Autodesk Fusion 360 part; units mm, degrees
(part 8 of 8)
  spline S41 degree 5 poles (20.6515, -12.2277) (20.6495, -12.2245) (20.6456, -12.2182) (20.6397, -12.2087) (20.6318, -12.1961) (20.6219, -12.1805) (20.6121, -12.1648) (20.6022, -12.1492) (20.5923, -12.1337) (20.5824, -12.1182) (20.5725, -12.1028) (20.5626, -12.0874) (20.5527, -12.0721) (20.5428, -12.0568) (20.5329, -12.0416) (20.523, -12.0264) (20.5131, -12.0112) (20.5032, -11.9962) (20.4932, -11.9811) (20.4833, -11.9661) (20.4734, -11.9512) (20.4634, -11.9363) (20.4535, -11.9215) (20.4436, -11.9067) (20.4336, -11.892) (20.4237, -11.8773) (20.4137, -11.8627) (20.4038, -11.8482) (20.3938, -11.8336) (20.3839, -11.8192) (20.3739, -11.8048) (20.364, -11.7904) (20.354, -11.7761) (20.3441, -11.7618) (20.3341, -11.7476) (20.3242, -11.7335) (20.3142, -11.7194) (20.3042, -11.7053) (20.2943, -11.6913) (20.2843, -11.6774) (20.2744, -11.6635) (20.2644, -11.6497) (20.2545, -11.6359) (20.2445, -11.6221) (20.2346, -11.6085) (20.2246, -11.5948) (20.2147, -11.5813) (20.2047, -11.5677) (20.1948, -11.5543) (20.1848, -11.5409) (20.1749, -11.5275) (20.165, -11.5142) (20.155, -11.501) (20.1451, -11.4878) (20.1352, -11.4746) (20.1253, -11.4615) (20.1154, -11.4485) (20.1054, -11.4355) (20.0955, -11.4226) (20.0856, -11.4097) (20.0757, -11.3969) (20.0659, -11.3842) (20.056, -11.3715) (20.0461, -11.3588) (20.0362, -11.3462) (20.0263, -11.3337) (20.0165, -11.3212) (20.0066, -11.3088) (19.9968, -11.2964) (19.9869, -11.2841) (19.9771, -11.2718) (19.9673, -11.2596) (19.9575, -11.2475) (19.9477, -11.2354) (19.9379, -11.2233) (19.9281, -11.2113) (19.9183, -11.1994) (19.9085, -11.1875) (19.8987, -11.1757) (19.889, -11.164) (19.8792, -11.1523) (19.8695, -11.1406) (19.8598, -11.1291) (19.8501, -11.1175) (19.8404, -11.1061) (19.8307, -11.0946) (19.821, -11.0833) (19.8113, -11.072) (19.8017, -11.0607) (19.7921, -11.0496) (19.7824, -11.0384) (19.7728, -11.0274) (19.7632, -11.0164) (19.7536, -11.0054) (19.7441, -10.9945) (19.7345, -10.9837) (19.725, -10.9729) (19.7154, -10.9622) (19.7059, -10.9515) (19.6964, -10.9409) (19.6869, -10.9304) (19.6775, -10.9199) (19.668, -10.9095) (19.6586, -10.8991) (19.6492, -10.8888) (19.6398, -10.8786) (19.6304, -10.8684) (19.621, -10.8583) (19.6117, -10.8482) (19.6024, -10.8382) (19.5931, -10.8282) (19.5838, -10.8184) (19.5745, -10.8085) (19.5653, -10.7988) (19.5561, -10.7891) (19.5469, -10.7794) (19.5377, -10.7698) (19.5285, -10.7603) (19.5194, -10.7509) (19.5103, -10.7415) (19.5012, -10.7321) (19.4921, -10.7229) (19.4831, -10.7136) (19.4741, -10.7045) (19.4651, -10.6954) (19.4561, -10.6864) (19.4472, -10.6774) (19.4382, -10.6685) (19.4293, -10.6596) (19.4205, -10.6509) (19.4116, -10.6421) (19.4028, -10.6335) (19.3941, -10.6249) (19.3853, -10.6164) (19.3766, -10.6079) (19.3679, -10.5995) (19.3592, -10.5912) (19.3506, -10.5829) (19.342, -10.5747) (19.3334, -10.5665) (19.3249, -10.5584) (19.3163, -10.5504) (19.3079, -10.5425) (19.2994, -10.5346) (19.291, -10.5267) (19.2826, -10.519) (19.2743, -10.5113) (19.266, -10.5036) (19.2577, -10.4961) (19.2495, -10.4886) (19.2413, -10.4811) (19.2331, -10.4738) (19.225, -10.4665) (19.2169, -10.4592) (19.2088, -10.452) (19.2008, -10.4449) (19.1929, -10.4379) (19.1849, -10.4309) (19.177, -10.424) (19.1692, -10.4172) (19.1614, -10.4104) (19.1536, -10.4037) (19.1459, -10.397) (19.1382, -10.3905) (19.1306, -10.384) (19.123, -10.3775) (19.1155, -10.3712) (19.108, -10.3649) (19.1006, -10.3586) (19.0932, -10.3525) (19.0858, -10.3464) (19.0785, -10.3403) (19.0713, -10.3344) (19.0641, -10.3285) (19.0569, -10.3227) (19.0498, -10.3169) (19.0428, -10.3112) (19.0358, -10.3056) (19.0289, -10.3001) (19.022, -10.2946) (19.0152, -10.2892) (19.0085, -10.2839) (19.0017, -10.2786) (18.9951, -10.2735) (18.9885, -10.2683) (18.982, -10.2633) (18.9755, -10.2583) (18.9691, -10.2534) (18.9628, -10.2486) (18.9565, -10.2439) (18.9503, -10.2392) (18.9442, -10.2346) (18.9381, -10.23) (18.9321, -10.2256) (18.9262, -10.2212) (18.9203, -10.2169) (18.9145, -10.2127) (18.9088, -10.2085) (18.9032, -10.2044) (18.8976, -10.2004) (18.8921, -10.1965) (18.8867, -10.1926) (18.8814, -10.1888) (18.8761, -10.1851) (18.8709, -10.1815) (18.8658, -10.1779) (18.8608, -10.1745) (18.8559, -10.1711) (18.8511, -10.1677) (18.8463, -10.1645) (18.8417, -10.1613) (18.8371, -10.1583) (18.8326, -10.1553) (18.8282, -10.1523) (18.824, -10.1495) (18.8198, -10.1467) (18.8157, -10.144) (18.8117, -10.1414) (18.8078, -10.1389) (18.804, -10.1365) (18.8003, -10.1341) (18.7968, -10.1319) (18.7933, -10.1297) (18.79, -10.1276) (18.7868, -10.1256) (18.7836, -10.1236) (18.7807, -10.1218) (18.7778, -10.12) (18.775, -10.1183) (18.7724, -10.1168) (18.7699, -10.1153) (18.7676, -10.1138) (18.7654, -10.1125) (18.7633, -10.1113) (18.7613, -10.1102) (18.7595, -10.1091) (18.7579, -10.1081) (18.7564, -10.1073) (18.755, -10.1065) (18.7538, -10.1058) (18.7528, -10.1053) (18.7521, -10.1049) (18.7517, -10.1046) (18.7514, -10.1045) (18.7513, -10.1044) knots -1 -1 -1 -1 -1 -1 -0.99583333 -0.99166667 -0.9875 -0.98333333 -0.97916667 -0.975 -0.97083333 -0.96666667 -0.9625 -0.95833333 -0.95416667 -0.95 -0.94583333 -0.94166667 -0.9375 -0.93333333 -0.92916667 -0.925 -0.92083333 -0.91666667 -0.9125 -0.90833333 -0.90416667 -0.9 -0.89583333 -0.89166667 -0.8875 -0.88333333 -0.87916667 -0.875 -0.87083333 -0.86666667 -0.8625 -0.85833333 -0.85416667 -0.85 -0.84583333 -0.84166667 -0.8375 -0.83333333 -0.82916667 -0.825 -0.82083333 -0.81666667 -0.8125 -0.80833333 -0.80416667 -0.8 -0.79583333 -0.79166667 -0.7875 -0.78333333 -0.77916667 -0.775 -0.77083333 -0.76666667 -0.7625 -0.75833333 -0.75416667 -0.75 -0.74583333 -0.74166667 -0.7375 -0.73333333 -0.72916667 -0.725 -0.72083333 -0.71666667 -0.7125 -0.70833333 -0.70416667 -0.7 -0.69583333 -0.69166667 -0.6875 -0.68333333 -0.67916667 -0.675 -0.67083333 -0.66666667 -0.6625 -0.65833333 -0.65416667 -0.65 -0.64583333 -0.64166667 -0.6375 -0.63333333 -0.62916667 -0.625 -0.62083333 -0.61666667 -0.6125 -0.60833333 -0.60416667 -0.6 -0.59583333 -0.59166667 -0.5875 -0.58333333 -0.57916667 -0.575 -0.57083333 -0.56666667 -0.5625 -0.55833333 -0.55416667 -0.55 -0.54583333 -0.54166667 -0.5375 -0.53333333 -0.52916667 -0.525 -0.52083333 -0.51666667 -0.5125 -0.50833333 -0.50416667 -0.5 -0.49583333 -0.49166667 -0.4875 -0.48333333 -0.47916667 -0.475 -0.47083333 -0.46666667 -0.4625 -0.45833333 -0.45416667 -0.45 -0.44583333 -0.44166667 -0.4375 -0.43333333 -0.42916667 -0.425 -0.42083333 -0.41666667 -0.4125 -0.40833333 -0.40416667 -0.4 -0.39583333 -0.39166667 -0.3875 -0.38333333 -0.37916667 -0.375 -0.37083333 -0.36666667 -0.3625 -0.35833333 -0.35416667 -0.35 -0.34583333 -0.34166667 -0.3375 -0.33333333 -0.32916667 -0.325 -0.32083333 -0.31666667 -0.3125 -0.30833333 -0.30416667 -0.3 -0.29583333 -0.29166667 -0.2875 -0.28333333 -0.27916667 -0.275 -0.27083333 -0.26666667 -0.2625 -0.25833333 -0.25416667 -0.25 -0.24583333 -0.24166667 -0.2375 -0.23333333 -0.22916667 -0.225 -0.22083333 -0.21666667 -0.2125 -0.20833333 -0.20416667 -0.2 -0.19583333 -0.19166667 -0.1875 -0.18333333 -0.17916667 -0.175 -0.17083333 -0.16666667 -0.1625 -0.15833333 -0.15416667 -0.15 -0.14583333 -0.14166667 -0.1375 -0.13333333 -0.12916667 -0.125 -0.12083333 -0.11666667 -0.1125 -0.10833333 -0.10416667 -0.1 -0.09583333 -0.09166667 -0.0875 -0.08333333 -0.07916667 -0.075 -0.07083333 -0.06666667 -0.0625 -0.05833333 -0.05416667 -0.05 -0.04583333 -0.04166667 -0.0375 -0.03333333 -0.02916667 -0.025 -0.02083333 -0.01666667 -0.0125 -0.00833333 -0.00416667 0 0 0 0 0 0
  line L82 (18.7513, -10.1044) -> (18.7502, -10.1038)
  line L83 (18.7502, -10.1038) -> (17.1663, -9.2503)
  arc A42 (17.1663, -9.2503) -> (18.2325, -6.9158) centre (0, 0) ccw
  line L84 (18.2325, -6.9158) -> (19.9147, -7.5539)
  line L85 (19.9147, -7.5539) -> (19.9159, -7.5543)
  spline S42 degree 5 poles (19.9159, -7.5543) (19.916, -7.5543) (19.9163, -7.5544) (19.9168, -7.5546) (19.9175, -7.5549) (19.9186, -7.5553) (19.9199, -7.5557) (19.9214, -7.5563) (19.923, -7.5568) (19.9248, -7.5574) (19.9268, -7.5581) (19.9289, -7.5588) (19.9312, -7.5596) (19.9337, -7.5604) (19.9363, -7.5613) (19.9391, -7.5622) (19.942, -7.5631) (19.945, -7.5641) (19.9482, -7.5651) (19.9516, -7.5662) (19.9551, -7.5673) (19.9587, -7.5684) (19.9625, -7.5695) (19.9664, -7.5707) (19.9705, -7.5719) (19.9747, -7.5731) (19.979, -7.5744) (19.9834, -7.5757) (19.988, -7.577) (19.9927, -7.5783) (19.9975, -7.5797) (20.0025, -7.5811) (20.0076, -7.5825) (20.0128, -7.5839) (20.0181, -7.5853) (20.0235, -7.5868) (20.0291, -7.5882) (20.0348, -7.5897) (20.0406, -7.5912) (20.0465, -7.5927) (20.0525, -7.5942) (20.0586, -7.5958) (20.0649, -7.5973) (20.0712, -7.5989) (20.0777, -7.6004) (20.0843, -7.602) (20.0909, -7.6036) (20.0977, -7.6052) (20.1046, -7.6068) (20.1116, -7.6084) (20.1187, -7.61) (20.1259, -7.6116) (20.1332, -7.6132) (20.1406, -7.6148) (20.1481, -7.6165) (20.1557, -7.6181) (20.1634, -7.6197) (20.1712, -7.6213) (20.1791, -7.623) (20.1871, -7.6246) (20.1951, -7.6262) (20.2033, -7.6279) (20.2116, -7.6295) (20.2199, -7.6311) (20.2284, -7.6327) (20.2369, -7.6343) (20.2456, -7.636) (20.2543, -7.6376) (20.2631, -7.6392) (20.272, -7.6408) (20.281, -7.6424) (20.2901, -7.644) (20.2992, -7.6455) (20.3085, -7.6471) (20.3178, -7.6487) (20.3272, -7.6502) (20.3367, -7.6518) (20.3463, -7.6533) (20.356, -7.6549) (20.3657, -7.6564) (20.3756, -7.6579) (20.3855, -7.6594) (20.3955, -7.6609) (20.4055, -7.6624) (20.4157, -7.6639) (20.4259, -7.6653) (20.4362, -7.6668) (20.4466, -7.6682) (20.4571, -7.6696) (20.4676, -7.671) (20.4782, -7.6724) (20.4889, -7.6738) (20.4997, -7.6752) (20.5105, -7.6765) (20.5215, -7.6779) (20.5325, -7.6792) (20.5435, -7.6805) (20.5547, -7.6818) (20.5659, -7.6831) (20.5771, -7.6844) (20.5885, -7.6856) (20.5999, -7.6868) (20.6114, -7.6881) (20.623, -7.6893) (20.6346, -7.6904) (20.6463, -7.6916) (20.6581, -7.6927) (20.6699, -7.6939) (20.6819, -7.695) (20.6938, -7.6961) (20.7059, -7.6971) (20.718, -7.6982) (20.7302, -7.6992) (20.7424, -7.7002) (20.7547, -7.7012) (20.7671, -7.7022) (20.7795, -7.7031) (20.792, -7.7041) (20.8046, -7.705) (20.8172, -7.7059) (20.8299, -7.7067) (20.8427, -7.7076) (20.8555, -7.7084) (20.8684, -7.7092) (20.8814, -7.71) (20.8944, -7.7107) (20.9074, -7.7115) (20.9206, -7.7122) (20.9338, -7.7128) (20.947, -7.7135) (20.9603, -7.7141) (20.9737, -7.7148) (20.9871, -7.7154) (21.0006, -7.7159) (21.0142, -7.7165) (21.0278, -7.717) (21.0415, -7.7175) (21.0552, -7.7179) (21.069, -7.7184) (21.0828, -7.7188) (21.0967, -7.7192) (21.1106, -7.7196) (21.1247, -7.7199) (21.1387, -7.7202) (21.1528, -7.7205) (21.167, -7.7208) (21.1812, -7.721) (21.1955, -7.7212) (21.2099, -7.7214) (21.2243, -7.7216) (21.2387, -7.7217) (21.2532, -7.7218) (21.2678, -7.7219) (21.2824, -7.7219) (21.297, -7.7219) (21.3117, -7.7219) (21.3265, -7.7219) (21.3413, -7.7218) (21.3562, -7.7217) (21.3711, -7.7216) (21.3861, -7.7214) (21.4011, -7.7213) (21.4162, -7.721) (21.4313, -7.7208) (21.4465, -7.7205) (21.4617, -7.7202) (21.477, -7.7199) (21.4923, -7.7196) (21.5077, -7.7192) (21.5231, -7.7188) (21.5385, -7.7183) (21.5541, -7.7178) (21.5696, -7.7173) (21.5852, -7.7168) (21.6009, -7.7162) (21.6166, -7.7156) (21.6323, -7.715) (21.6481, -7.7143) (21.664, -7.7136) (21.6799, -7.7129) (21.6958, -7.7122) (21.7118, -7.7114) (21.7278, -7.7106) (21.7439, -7.7097) (21.76, -7.7088) (21.7762, -7.7079) (21.7924, -7.707) (21.8087, -7.706) (21.825, -7.705) (21.8413, -7.704) (21.8577, -7.7029) (21.8741, -7.7018) (21.8906, -7.7006) (21.9071, -7.6995) (21.9237, -7.6983) (21.9403, -7.697) (21.9569, -7.6958) (21.9736, -7.6945) (21.9903, -7.6931) (22.0071, -7.6917) (22.0239, -7.6903) (22.0408, -7.6889) (22.0577, -7.6874) (22.0746, -7.6859) (22.0916, -7.6844) (22.1086, -7.6828) (22.1256, -7.6812) (22.1427, -7.6796) (22.1599, -7.6779) (22.1771, -7.6762) (22.1943, -7.6744) (22.2115, -7.6727) (22.2288, -7.6708) (22.2462, -7.669) (22.2635, -7.6671) (22.2809, -7.6652) (22.2984, -7.6632) (22.3159, -7.6613) (22.3334, -7.6592) (22.351, -7.6572) (22.3686, -7.6551) (22.3862, -7.653) (22.4039, -7.6508) (22.4216, -7.6486) (22.4393, -7.6464) (22.4571, -7.6441) (22.4749, -7.6418) (22.4928, -7.6394) (22.5107, -7.6371) (22.5286, -7.6347) (22.5466, -7.6322) (22.5646, -7.6297) (22.5826, -7.6272) (22.6007, -7.6246) (22.6188, -7.622) (22.637, -7.6194) (22.6551, -7.6167) (22.6733, -7.614) (22.6916, -7.6113) (22.7099, -7.6085) (22.7282, -7.6057) (22.7428, -7.6034) (22.7539, -7.6017) (22.7612, -7.6005) (22.7649, -7.5999) knots 0 0 0 0 0 0 0.00416667 0.00833333 0.0125 0.01666667 0.02083333 0.025 0.02916667 0.03333333 0.0375 0.04166667 0.04583333 0.05 0.05416667 0.05833333 0.0625 0.06666667 0.07083333 0.075 0.07916667 0.08333333 0.0875 0.09166667 0.09583333 0.1 0.10416667 0.10833333 0.1125 0.11666667 0.12083333 0.125 0.12916667 0.13333333 0.1375 0.14166667 0.14583333 0.15 0.15416667 0.15833333 0.1625 0.16666667 0.17083333 0.175 0.17916667 0.18333333 0.1875 0.19166667 0.19583333 0.2 0.20416667 0.20833333 0.2125 0.21666667 0.22083333 0.225 0.22916667 0.23333333 0.2375 0.24166667 0.24583333 0.25 0.25416667 0.25833333 0.2625 0.26666667 0.27083333 0.275 0.27916667 0.28333333 0.2875 0.29166667 0.29583333 0.3 0.30416667 0.30833333 0.3125 0.31666667 0.32083333 0.325 0.32916667 0.33333333 0.3375 0.34166667 0.34583333 0.35 0.35416667 0.35833333 0.3625 0.36666667 0.37083333 0.375 0.37916667 0.38333333 0.3875 0.39166667 0.39583333 0.4 0.40416667 0.40833333 0.4125 0.41666667 0.42083333 0.425 0.42916667 0.43333333 0.4375 0.44166667 0.44583333 0.45 0.45416667 0.45833333 0.4625 0.46666667 0.47083333 0.475 0.47916667 0.48333333 0.4875 0.49166667 0.49583333 0.5 0.50416667 0.50833333 0.5125 0.51666667 0.52083333 0.525 0.52916667 0.53333333 0.5375 0.54166667 0.54583333 0.55 0.55416667 0.55833333 0.5625 0.56666667 0.57083333 0.575 0.57916667 0.58333333 0.5875 0.59166667 0.59583333 0.6 0.60416667 0.60833333 0.6125 0.61666667 0.62083333 0.625 0.62916667 0.63333333 0.6375 0.64166667 0.64583333 0.65 0.65416667 0.65833333 0.6625 0.66666667 0.67083333 0.675 0.67916667 0.68333333 0.6875 0.69166667 0.69583333 0.7 0.70416667 0.70833333 0.7125 0.71666667 0.72083333 0.725 0.72916667 0.73333333 0.7375 0.74166667 0.74583333 0.75 0.75416667 0.75833333 0.7625 0.76666667 0.77083333 0.775 0.77916667 0.78333333 0.7875 0.79166667 0.79583333 0.8 0.80416667 0.80833333 0.8125 0.81666667 0.82083333 0.825 0.82916667 0.83333333 0.8375 0.84166667 0.84583333 0.85 0.85416667 0.85833333 0.8625 0.86666667 0.87083333 0.875 0.87916667 0.88333333 0.8875 0.89166667 0.89583333 0.9 0.90416667 0.90833333 0.9125 0.91666667 0.92083333 0.925 0.92916667 0.93333333 0.9375 0.94166667 0.94583333 0.95 0.95416667 0.95833333 0.9625 0.96666667 0.97083333 0.975 0.97916667 0.98333333 0.9875 0.99166667 0.99583333 1 1 1 1 1 1
  arc A43 (22.7649, -7.5999) -> (23.2599, -5.9142) centre (0, 0) ccw
  spline S43 degree 5 poles (23.2599, -5.9142) (23.2571, -5.9117) (23.2516, -5.9067) (23.2432, -5.8993) (23.2321, -5.8895) (23.2182, -5.8772) (23.2043, -5.865) (23.1905, -5.8528) (23.1766, -5.8407) (23.1628, -5.8286) (23.1489, -5.8166) (23.1351, -5.8046) (23.1213, -5.7927) (23.1075, -5.7808) (23.0937, -5.769) (23.0799, -5.7572) (23.0661, -5.7455) (23.0523, -5.7338) (23.0386, -5.7222) (23.0248, -5.7106) (23.0111, -5.6991) (22.9974, -5.6876) (22.9837, -5.6762) (22.97, -5.6648) (22.9563, -5.6535) (22.9426, -5.6422) (22.929, -5.631) (22.9153, -5.6198) (22.9017, -5.6087) (22.888, -5.5976) (22.8744, -5.5866) (22.8608, -5.5756) (22.8473, -5.5647) (22.8337, -5.5538) (22.8201, -5.543) (22.8066, -5.5322) (22.7931, -5.5215) (22.7795, -5.5108) (22.7661, -5.5002) (22.7526, -5.4896) (22.7391, -5.4791) (22.7257, -5.4686) (22.7122, -5.4582) (22.6988, -5.4478) (22.6854, -5.4375) (22.672, -5.4272) (22.6587, -5.417) (22.6453, -5.4068) (22.632, -5.3967) (22.6187, -5.3867) (22.6054, -5.3766) (22.5921, -5.3667) (22.5788, -5.3568) (22.5656, -5.3469) (22.5524, -5.3371) (22.5391, -5.3273) (22.526, -5.3176) (22.5128, -5.3079) (22.4996, -5.2983) (22.4865, -5.2888) (22.4734, -5.2793) (22.4603, -5.2698) (22.4473, -5.2604) (22.4342, -5.2511) (22.4212, -5.2418) (22.4082, -5.2325) (22.3952, -5.2233) (22.3823, -5.2142) (22.3693, -5.2051) (22.3564, -5.196) (22.3435, -5.187) (22.3307, -5.1781) (22.3178, -5.1692) (22.305, -5.1603) (22.2922, -5.1516) (22.2794, -5.1428) (22.2667, -5.1341) (22.254, -5.1255) (22.2413, -5.1169) (22.2286, -5.1084) (22.216, -5.0999) (22.2033, -5.0915) (22.1907, -5.0831) (22.1782, -5.0748) (22.1656, -5.0665) (22.1531, -5.0583) (22.1406, -5.0501) (22.1282, -5.042) (22.1158, -5.0339) (22.1034, -5.0259) (22.091, -5.018) (22.0786, -5.01) (22.0663, -5.0022) (22.0541, -4.9944) (22.0418, -4.9866) (22.0296, -4.9789) (22.0174, -4.9713) (22.0052, -4.9637) (21.9931, -4.9561) (21.981, -4.9486) (21.9689, -4.9412) (21.9569, -4.9338) (21.9449, -4.9265) (21.9329, -4.9192) (21.921, -4.9119) (21.9091, -4.9048) (21.8972, -4.8976) (21.8854, -4.8905) (21.8736, -4.8835) (21.8618, -4.8765) (21.8501, -4.8696) (21.8384, -4.8628) (21.8267, -4.8559) (21.8151, -4.8492) (21.8035, -4.8425) (21.792, -4.8358) (21.7805, -4.8292) (21.769, -4.8226) (21.7576, -4.8161) (21.7462, -4.8097) (21.7348, -4.8033) (21.7235, -4.7969) (21.7123, -4.7906) (21.701, -4.7844) (21.6898, -4.7782) (21.6787, -4.7721) (21.6676, -4.766) (21.6565, -4.76) (21.6455, -4.754) (21.6345, -4.748) (21.6236, -4.7422) (21.6127, -4.7364) (21.6018, -4.7306) (21.591, -4.7249) (21.5803, -4.7192) (21.5696, -4.7136) (21.5589, -4.708) (21.5483, -4.7025) (21.5377, -4.6971) (21.5272, -4.6917) (21.5167, -4.6863) (21.5063, -4.681) (21.4959, -4.6758) (21.4856, -4.6706) (21.4753, -4.6654) (21.4651, -4.6603) (21.4549, -4.6553) (21.4448, -4.6503) (21.4347, -4.6454) (21.4247, -4.6405) (21.4147, -4.6357) (21.4048, -4.6309) (21.395, -4.6262) (21.3852, -4.6215) (21.3754, -4.6169) (21.3657, -4.6123) (21.3561, -4.6078) (21.3465, -4.6034) (21.337, -4.599) (21.3276, -4.5946) (21.3182, -4.5903) (21.3088, -4.5861) (21.2996, -4.5819) (21.2903, -4.5777) (21.2812, -4.5736) (21.2721, -4.5696) (21.2631, -4.5656) (21.2541, -4.5617) (21.2452, -4.5578) (21.2364, -4.5539) (21.2276, -4.5502) (21.2189, -4.5464) (21.2103, -4.5428) (21.2017, -4.5391) (21.1932, -4.5356) (21.1848, -4.5321) (21.1765, -4.5286) (21.1682, -4.5252) (21.16, -4.5218) (21.1518, -4.5185) (21.1438, -4.5152) (21.1358, -4.512) (21.1279, -4.5089) (21.12, -4.5058) (21.1123, -4.5027) (21.1046, -4.4997) (21.097, -4.4968) (21.0895, -4.4939) (21.0821, -4.491) (21.0747, -4.4882) (21.0674, -4.4855) (21.0602, -4.4828) (21.0531, -4.4802) (21.0461, -4.4776) (21.0392, -4.4751) (21.0324, -4.4726) (21.0256, -4.4701) (21.0189, -4.4678) (21.0124, -4.4654) (21.0059, -4.4631) (20.9995, -4.4609) (20.9932, -4.4587) (20.9871, -4.4566) (20.981, -4.4545) (20.975, -4.4525) (20.9691, -4.4505) (20.9633, -4.4486) (20.9576, -4.4467) (20.9521, -4.4449) (20.9466, -4.4431) (20.9412, -4.4414) (20.936, -4.4398) (20.9308, -4.4381) (20.9258, -4.4366) (20.9209, -4.435) (20.9161, -4.4336) (20.9114, -4.4321) (20.9069, -4.4308) (20.9024, -4.4295) (20.8981, -4.4282) (20.8939, -4.427) (20.8899, -4.4258) (20.8859, -4.4247) (20.8821, -4.4236) (20.8785, -4.4226) (20.8749, -4.4216) (20.8715, -4.4206) (20.8683, -4.4198) (20.8652, -4.4189) (20.8622, -4.4181) (20.8594, -4.4174) (20.8568, -4.4167) (20.8543, -4.4161) (20.8519, -4.4155) (20.8497, -4.4149) (20.8477, -4.4144) (20.8458, -4.414) (20.8441, -4.4136) (20.8426, -4.4132) (20.8413, -4.4129) (20.8402, -4.4126) (20.8394, -4.4125) (20.8389, -4.4124) (20.8386, -4.4123) (20.8384, -4.4123) knots -1 -1 -1 -1 -1 -1 -0.99583333 -0.99166667 -0.9875 -0.98333333 -0.97916667 -0.975 -0.97083333 -0.96666667 -0.9625 -0.95833333 -0.95416667 -0.95 -0.94583333 -0.94166667 -0.9375 -0.93333333 -0.92916667 -0.925 -0.92083333 -0.91666667 -0.9125 -0.90833333 -0.90416667 -0.9 -0.89583333 -0.89166667 -0.8875 -0.88333333 -0.87916667 -0.875 -0.87083333 -0.86666667 -0.8625 -0.85833333 -0.85416667 -0.85 -0.84583333 -0.84166667 -0.8375 -0.83333333 -0.82916667 -0.825 -0.82083333 -0.81666667 -0.8125 -0.80833333 -0.80416667 -0.8 -0.79583333 -0.79166667 -0.7875 -0.78333333 -0.77916667 -0.775 -0.77083333 -0.76666667 -0.7625 -0.75833333 -0.75416667 -0.75 -0.74583333 -0.74166667 -0.7375 -0.73333333 -0.72916667 -0.725 -0.72083333 -0.71666667 -0.7125 -0.70833333 -0.70416667 -0.7 -0.69583333 -0.69166667 -0.6875 -0.68333333 -0.67916667 -0.675 -0.67083333 -0.66666667 -0.6625 -0.65833333 -0.65416667 -0.65 -0.64583333 -0.64166667 -0.6375 -0.63333333 -0.62916667 -0.625 -0.62083333 -0.61666667 -0.6125 -0.60833333 -0.60416667 -0.6 -0.59583333 -0.59166667 -0.5875 -0.58333333 -0.57916667 -0.575 -0.57083333 -0.56666667 -0.5625 -0.55833333 -0.55416667 -0.55 -0.54583333 -0.54166667 -0.5375 -0.53333333 -0.52916667 -0.525 -0.52083333 -0.51666667 -0.5125 -0.50833333 -0.50416667 -0.5 -0.49583333 -0.49166667 -0.4875 -0.48333333 -0.47916667 -0.475 -0.47083333 -0.46666667 -0.4625 -0.45833333 -0.45416667 -0.45 -0.44583333 -0.44166667 -0.4375 -0.43333333 -0.42916667 -0.425 -0.42083333 -0.41666667 -0.4125 -0.40833333 -0.40416667 -0.4 -0.39583333 -0.39166667 -0.3875 -0.38333333 -0.37916667 -0.375 -0.37083333 -0.36666667 -0.3625 -0.35833333 -0.35416667 -0.35 -0.34583333 -0.34166667 -0.3375 -0.33333333 -0.32916667 -0.325 -0.32083333 -0.31666667 -0.3125 -0.30833333 -0.30416667 -0.3 -0.29583333 -0.29166667 -0.2875 -0.28333333 -0.27916667 -0.275 -0.27083333 -0.26666667 -0.2625 -0.25833333 -0.25416667 -0.25 -0.24583333 -0.24166667 -0.2375 -0.23333333 -0.22916667 -0.225 -0.22083333 -0.21666667 -0.2125 -0.20833333 -0.20416667 -0.2 -0.19583333 -0.19166667 -0.1875 -0.18333333 -0.17916667 -0.175 -0.17083333 -0.16666667 -0.1625 -0.15833333 -0.15416667 -0.15 -0.14583333 -0.14166667 -0.1375 -0.13333333 -0.12916667 -0.125 -0.12083333 -0.11666667 -0.1125 -0.10833333 -0.10416667 -0.1 -0.09583333 -0.09166667 -0.0875 -0.08333333 -0.07916667 -0.075 -0.07083333 -0.06666667 -0.0625 -0.05833333 -0.05416667 -0.05 -0.04583333 -0.04166667 -0.0375 -0.03333333 -0.02916667 -0.025 -0.02083333 -0.01666667 -0.0125 -0.00833333 -0.00416667 0 0 0 0 0 0
  line L86 (20.8384, -4.4123) -> (20.8373, -4.412)
  line L87 (20.8373, -4.412) -> (19.0771, -4.0393)
  line L88 (18, -3) -> (-18, -3)
  line L89 (-18, -3) -> (-18, 3)
  line L90 (-18, 3) -> (18, 3)
  line L91 (18, 3) -> (18, -3)
  line L92 (18, -3) -> (-18, 3) construction
  line L93 (-18, -3) -> (18, 3) construction
  dimension "d31" = 36
  dimension "d32" = 6
  constraint horizontal L88
  constraint perpendicular L88 L89
  constraint parallel L88 L90
  constraint parallel L89 L91
  constraint coincident L92 A0.centre
  constraint coincident L93 A0.centre
  constraint coincident A0.centre A1.centre
  measures "d31" distance of L89.end L90.end
  measures "d32" distance of L88.end L89.end
extrude "Extrude3" cut sketch "Sketch1 (2)" against normal blind 2 contours L88 L89 L90 L91 bodies 1 in component "Component"
extrude "Extrude4" cut 1 faces at (-2.8242, 3.262, 0) along direction (0, 0, 1) blind 5 on bodies 1 bodies 1 in component "Component"
component "Component" placed x (1, 0, 0) y (0, 1, 0) z (0, 0, 1) at (0, 0, 0)
